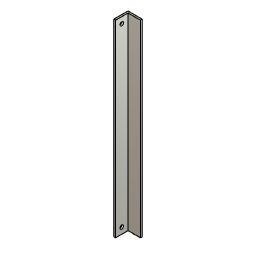
Middle Platform Assembly v15 (Autodesk Fusion 360 archive; units mm, degrees)
design "Angle 336.4 mm 2nd 3rd FR"
Autodesk Fusion 360 part; units mm, degrees
note: some values were not read from the file. Chosen so that the rebuilt part matches the saved one: which bodies a step acts on; a direction. Set by a fixed rule: which sketch regions a step uses.
sketch "Sketch1" plane through (0, 0, 0) normal (0, 1, 0) x (1, 0, 0)
  line L0 (0, -25.4) -> (0, 0)
  line L1 (0, 0) -> (25.4, 0)
  line L2 (12.7, -12.7) -> (11.05, -11.05) construction
  line L3 (3.175, -25.4) -> (3.175, -3.175)
  line L4 (3.175, -3.175) -> (25.4, -3.175)
  line L5 (25.4, -3.175) -> (25.4, 0)
  line L6 (0, -25.4) -> (3.175, -25.4)
  dimension "d1" = 25.4
  dimension "d2" = 25.4
  dimension "d13" = 3.175
  constraint coincident L0.end L2
  constraint coincident L0.end L1.start
  constraint perpendicular L1 L5
  constraint vertical L0
  constraint horizontal L1
  measures "d1" distance of L0.end L1.end
  measures "d2" distance of L0.start L0.end
extrude "Extrude1" add sketch "Sketch1" along normal blind 168.2
hole "Hole3" at (3.175, 157.087, 14.2875) direction (-1, 0, 0) diameter 6.5 end through all
mirror "Mirror1" about plane through (0, 0, 0) normal (0, 1, 0) of bodies 1 merged
equation "d5 = ( 336.4 / 2 ) * 1 mm"
equation "d27 = ( 22.225 / 2 ) * 1 mm"
equation "d19 = 25.4 mm - 11.113 mm"

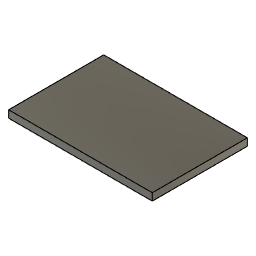
design "Razer 15 inch"
Autodesk Fusion 360 part; units mm, degrees
sketch "Sketch1" plane through (0, 0, 0) normal (0, 0, 1) x (1, 0, 0)
  line L0 (177.5, -117.5) -> (-177.5, -117.5)
  line L1 (-177.5, -117.5) -> (-177.5, 117.5)
  line L2 (-177.5, 117.5) -> (177.5, 117.5)
  line L3 (177.5, 117.5) -> (177.5, -117.5)
  line L4 (177.5, -117.5) -> (-177.5, 117.5) construction
  line L5 (-177.5, -117.5) -> (177.5, 117.5) construction
  dimension "d1" = 355
  dimension "d2" = 235
  constraint horizontal L0
  constraint perpendicular L0 L1
  constraint parallel L0 L2
  constraint parallel L1 L3
  constraint coincident L4 origin
  constraint coincident L5 origin
  measures "d1" distance of L1.end L2.end
  measures "d2" distance of L0.end L1.end
extrude "Extrude1" add sketch "Sketch1" along normal blind 18

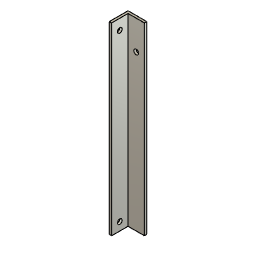
design "Angle 250 mm 1st Standing"
Autodesk Fusion 360 part; units mm, degrees
sketch "Sketch1" plane through (0, 0, 0) normal (0, 1, 0) x (1, 0, 0)
  line L0 (0, -25.4) -> (0, 0)
  line L1 (0, 0) -> (25.4, 0)
  line L2 (12.7, -12.7) -> (11.05, -11.05) construction
  line L3 (3.175, -25.4) -> (3.175, -3.175)
  line L4 (3.175, -3.175) -> (25.4, -3.175)
  line L5 (25.4, -3.175) -> (25.4, 0)
  line L6 (0, -25.4) -> (3.175, -25.4)
  dimension "d1" = 25.4
  dimension "d2" = 25.4
  dimension "d13" = 3.175
  constraint coincident L0.end L2
  constraint coincident L0.end L1.start
  constraint perpendicular L1 L5
  constraint perpendicular L0 L1
  constraint vertical L0
  measures "d1" distance of L0.end L1.end
  measures "d2" distance of L0.start L0.end
extrude "Extrude1" add sketch "Sketch1" along normal blind 250
sketch "Sketch2" plane through (3.175, 0, 0) normal (1, 0, 0) x (0, 0, -1)
  line L0 (-25.4, 0) -> (-3.175, 0)
  line L1 (-3.175, 0) -> (-3.175, 250)
  line L2 (-3.175, 250) -> (-25.4, 250)
  line L3 (-25.4, 250) -> (-25.4, 0)
  circle A0 centre (-14.2875, 235.712) radius 2.76
  circle A1 centre (-14.2875, 11.1125) radius 2.5546
  line L4 (-14.2875, 250) -> (-14.2875, 0) construction
  dimension "d14" = 14.288
  dimension "d15" = 11.1125
  constraint vertical A0.centre A1.centre
  constraint midpoint L2 L4.start
  constraint midpoint L0 L4.end
  constraint coincident A1.centre L4
  measures "d14" distance of L2 A0.centre
  measures "d15" distance of L0 A1.centre
hole "Hole1" at (3.175, 11.1125, 14.2875) at (3.175, 235.712, 14.2875) direction (-1, 0, 0) diameter 6.5 end through all
hole "Hole2" at (14.287, 210.312, 3.175) direction (0, 0, -1) diameter 6.5 end through all
equation "d15 = ( 22.225 / 2 ) * 1 mm"

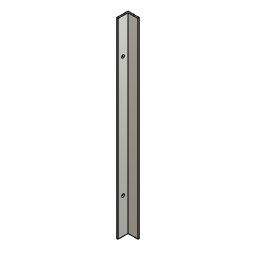
design "Angle 430 mm 2nd Side"
Autodesk Fusion 360 part; units mm, degrees
sketch "Sketch1" plane through (0, 0, 0) normal (0, 1, 0) x (1, 0, 0)
  line L0 (0, -25.4) -> (0, 0)
  line L1 (0, 0) -> (25.4, 0)
  line L2 (12.7, -12.7) -> (11.05, -11.05) construction
  line L3 (3.175, -25.4) -> (3.175, -3.175)
  line L4 (3.175, -3.175) -> (25.4, -3.175)
  line L5 (25.4, -3.175) -> (25.4, 0)
  line L6 (0, -25.4) -> (3.175, -25.4)
  dimension "d1" = 25.4
  dimension "d2" = 25.4
  dimension "d13" = 3.175
  constraint coincident L0.end L2
  constraint coincident L0.end L1.start
  constraint perpendicular L1 L5
  constraint vertical L0
  constraint horizontal L1
  measures "d1" distance of L0.end L1.end
  measures "d2" distance of L0.start L0.end
extrude "Extrude1" add sketch "Sketch1" along normal blind 215
hole "Hole3" at (3.175, 135.512, 14.2875) direction (-1, 0, 0) diameter 6.5 end through all
mirror "Mirror1" about plane through (0, 0, 0) normal (0, 1, 0) of bodies 1 merged
equation "d5 = ( 430 / 2 ) * 1 mm"
equation "d27 = ( 22.225 / 2 ) * 1 mm"
equation "d19 = 25.4 mm - 11.113 mm"

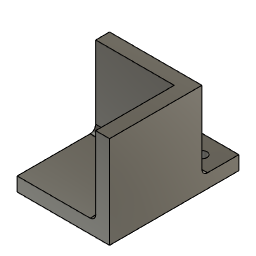
design "Laptop Mount RL/FR"
Autodesk Fusion 360 part; units mm, degrees
sketch "Sketch1" plane through (0, 0, 0) normal (0, 0, 1) x (1, 0, 0)
  line L0 (0, 0) -> (50, 0)
  line L1 (50, 0) -> (50, 50)
  line L2 (0, 7.5) -> (42.5, 7.5)
  line L3 (42.5, 7.5) -> (42.5, 50)
  line L4 (0, 7.5) -> (0, 0)
  line L5 (42.5, 50) -> (50, 50)
  dimension "d1" = -7.5
  dimension "d2" = 50
  dimension "d3" = 50
  constraint coincident L0.start L4.end
  constraint horizontal L0
  constraint perpendicular L0 L1
  constraint perpendicular L2 L4
  constraint perpendicular L1 L5
  measures "d2" distance of L0.start L0.end
  measures "d3" distance of L0.end L1.end
extrude "Extrude1" add sketch "Sketch1" along normal blind 50 makes body 1
sketch "Sketch4" plane through (0, 0, 0) normal (0, 0, 1) x (1, 0, 0)
  line L0 (0, -20) -> (50, -20)
  line L1 (50, -20) -> (50, 50)
  line L2 (50, 50) -> (0, 50)
  line L3 (0, 50) -> (0, -20)
  point P0 (50, 50)
  dimension "d43" = 70
  dimension "d44" = 50
  constraint horizontal L0
  constraint vertical L1
  constraint horizontal L2
  constraint vertical L3
  constraint coincident P0 L1.end
  measures "d43" distance of L0.start L2.end
  measures "d44" distance of P0 L2.end
extrude "Extrude4" add sketch "Sketch4" along normal blind 7.5 bodies 1
sketch "Sketch7" plane through (0, 0, 7.5) normal (0, 0, 1) x (-1, 0, 0)
  line L0 (-50, 20) -> (-50, 0)
  line L1 (0, 0) -> (0, 20)
  line L2 (-50, 0) -> (0, 0)
  line L3 (0, 20) -> (-50, 20)
  point P0 (-10, 10)
  point P1 (-40, 10)
  dimension "d30" = 10
  dimension "d31" = 30
  measures "d30" distance of L1 P0
  measures "d31" distance of P0 P1
hole "Hole1" at (10, -10, 7.5) at (40, -10, 7.5) direction (0, 0, -1) diameter 5.5 depth 10 tip angle 118 bodies 1
ref_plane "WorkPlane1" through (46.25, 50, 25) normal (0, 1, 0) x (-1, 0, 0)
mirror "Mirror1" about plane through (46.25, 50, 25) normal (0, 1, 0) of bodies 1 merged
split "Split1" by plane through (46.25, 50, 25) normal (0, 1, 0) bodies 1 makes body 2 at (29.6023, 69.1741, 0)
fillet "Fillet2" radius 3 3 edges at (25, 100, 7.5) (21.25, 92.5, 7.5) (42.5, 71.25, 7.5) on bodies 2
hidden bodies 1

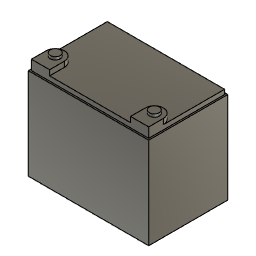
design "Battery"
Autodesk Fusion 360 part; units mm, degrees
sketch "Sketch1" plane through (0, 0, 0) normal (0, 0, 1) x (1, 0, 0)
  line L0 (96, -63) -> (-96, -63)
  line L1 (-96, -63) -> (-96, 63)
  line L2 (-96, 63) -> (96, 63)
  line L3 (96, 63) -> (96, -63)
  line L4 (96, -63) -> (-96, 63) construction
  line L5 (-96, -63) -> (96, 63) construction
  dimension "d1" = 192
  dimension "d2" = 126
  constraint horizontal L0
  constraint perpendicular L0 L1
  constraint parallel L0 L2
  constraint parallel L1 L3
  constraint coincident L4 origin
  constraint coincident L5 origin
  measures "d1" distance of L1.end L2.end
  measures "d2" distance of L0.end L1.end
extrude "Extrude1" add sketch "Sketch1" along normal blind 145.75
sketch "Sketch4" plane through (0, 0, 145.75) normal (0, 0, 1) x (-1, 0, 0)
  line L0 (-96, -63) -> (96, -63)
  line L1 (96, -63) -> (96, 63)
  line L2 (96, 63) -> (-96, 63)
  line L3 (-96, 63) -> (-96, -63)
  line L4 (96, -63) -> (-96, -63)
  line L5 (-96, -63) -> (-96, 63)
  line L6 (-96, 63) -> (96, 63)
  line L7 (96, 63) -> (96, -63)
  line L8 (-93.5, 60.5) -> (93.5, 60.5)
  line L9 (93.5, 60.5) -> (93.5, -60.5)
  line L10 (93.5, -60.5) -> (-93.5, -60.5)
  line L11 (-93.5, -60.5) -> (-93.5, 60.5)
  dimension "d12" = 2.5
  constraint horizontal L4
  constraint vertical L5
  constraint horizontal L6
  constraint vertical L7
  constraint coincident L2.end L3.start
  constraint coincident L0.end L1.start
extrude "Extrude4" add sketch "Sketch4" along normal blind 7.25 contours L8 L9 L10 L11
sketch "Sketch5" plane through (0, 0, 153) normal (0, 0, 1) x (-1, 0, 0)
  line L0 (-93.5, -60.5) -> (93.5, -60.5)
  line L1 (93.5, -60.5) -> (93.5, 60.5)
  line L2 (93.5, 60.5) -> (-93.5, 60.5)
  line L3 (-93.5, 60.5) -> (-93.5, -60.5)
  line L4 (93.5, 60.5) -> (64.5, 60.5)
  line L5 (64.5, 60.5) -> (64.5, 37)
  line L6 (93.5, 37) -> (93.5, 60.5)
  line L7 (-93.5, 60.5) -> (-64.5, 60.5)
  line L8 (-64.5, 60.5) -> (-64.5, 37)
  line L9 (-93.5, 37) -> (-93.5, 60.5)
  arc A0 (64.5, 37) -> (93.5, 37) centre (79, 37) ccw
  arc A1 (-93.5, 37) -> (-64.5, 37) centre (-79, 37) ccw
  dimension "d15" = 14.5
  dimension "d16" = 23.5
  constraint horizontal L4
  constraint vertical L5
  constraint vertical L6
  constraint coincident L1.end L2.start
  constraint horizontal L7
  constraint vertical L8
  constraint vertical L9
  constraint coincident L2.end L3.start
  constraint tangent L6 A0
  constraint tangent L5 A0
  constraint tangent L8 A1
  constraint tangent L9 A1
  constraint equal A0 A1
  constraint equal L5 L8
  measures "d15" radius of A0
  measures "d16" distance of L4.end L5.end
extrude "Extrude5" add sketch "Sketch5" along normal blind 8.5 contours L2 L3 L7 L8 L9 A1 | L1 L2 L4 L5 L6 A0
sketch "Sketch6" plane through (0, 0, 161.5) normal (0, 0, 1) x (-1, 0, 0)
  arc A0 (64.5, 37) -> (93.5, 37) centre (79, 37) ccw
  line L0 (93.5, 37) -> (93.5, 60.5)
  line L1 (93.5, 60.5) -> (64.5, 60.5)
  line L2 (64.5, 60.5) -> (64.5, 37)
  circle A1 centre (79, 37) radius 8
  circle A2 centre (-79, 37) radius 8
  arc A3 (-93.5, 37) -> (-64.5, 37) centre (-79, 37) ccw
  dimension "d19" = 16
  constraint concentric A0 A1
  constraint concentric A2 A3
  constraint equal A1 A2
  measures "d19" diameter of A1
extrude "Extrude6" add sketch "Sketch6" along normal blind 4.6 contours A1 | A2
equation "d3 = 153 mm - 7.25 mm"
equation "d16 = 38 mm - 14.5 mm"

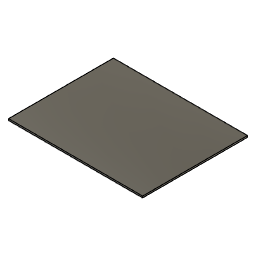
design "2nd Plate M"
Autodesk Fusion 360 part; units mm, degrees
sketch "Sketch1" plane through (0, 0, 0) normal (0, 0, 1) x (1, 0, 0)
  line L0 (-250, 225) -> (180, 225)
  line L1 (180, 225) -> (180, -111.4)
  line L2 (180, -111.4) -> (-250, -111.4)
  line L3 (-250, -111.4) -> (-250, 225)
  dimension "d1" = 336.4
  dimension "d2" = 430
  constraint horizontal L0
  constraint vertical L1
  constraint horizontal L2
  constraint vertical L3
  measures "d1" distance of L0.start L2.end
  measures "d2" distance of L0.start L0.end
extrude "Extrude1" add sketch "Sketch1" along normal blind 5

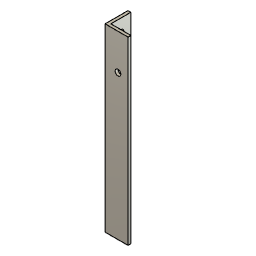
design "Angle 200 mm 2nd Standing Reverse"
Autodesk Fusion 360 part; units mm, degrees
sketch "Sketch1" plane through (0, 0, 0) normal (0, 1, 0) x (1, 0, 0)
  line L0 (0, -25.4) -> (0, 0)
  line L1 (0, 0) -> (25.4, 0)
  line L2 (12.7, -12.7) -> (11.05, -11.05) construction
  line L3 (3.175, -25.4) -> (3.175, -3.175)
  line L4 (3.175, -3.175) -> (25.4, -3.175)
  line L5 (25.4, -3.175) -> (25.4, 0)
  line L6 (0, -25.4) -> (3.175, -25.4)
  dimension "d1" = 25.4
  dimension "d2" = 25.4
  dimension "d13" = 3.175
  constraint coincident L0.end L2
  constraint coincident L0.end L1.start
  constraint perpendicular L1 L5
  constraint vertical L0
  constraint horizontal L1
  measures "d1" distance of L0.end L1.end
  measures "d2" distance of L0.start L0.end
extrude "Extrude1" add sketch "Sketch1" along normal blind 200 makes body 1
hole "Hole3" at (3.175, 11.113, 14.287) direction (-1, 0, 0) diameter 6.5 end through all bodies 1
hole "Hole4" at (3.175, 185.772, 14.287) direction (-1, 0, 0) diameter 6.5 depth 30 tip angle 118 bodies 1
hole "Hole5" at (14.287, 160.312, 3.175) direction (0, 0, -1) diameter 6.5 depth 30 tip angle 118 bodies 1
mirror "Mirror2" about plane through (0, 0, 0) normal (0, 0, -1) of bodies 1 makes body 2
delete_body "RemoveBody1" bodies 1

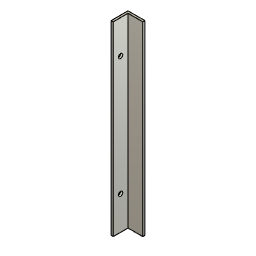
design "Angle 280 mm Battery Holder"
Autodesk Fusion 360 part; units mm, degrees
sketch "Sketch1" plane through (0, 0, 0) normal (0, 1, 0) x (1, 0, 0)
  line L0 (0, -25.4) -> (0, 0)
  line L1 (0, 0) -> (25.4, 0)
  line L2 (12.7, -12.7) -> (11.05, -11.05) construction
  line L3 (3.175, -25.4) -> (3.175, -3.175)
  line L4 (3.175, -3.175) -> (25.4, -3.175)
  line L5 (25.4, -3.175) -> (25.4, 0)
  line L6 (0, -25.4) -> (3.175, -25.4)
  dimension "d1" = 25.4
  dimension "d2" = 25.4
  dimension "d13" = 3.175
  constraint coincident L0.end L2
  constraint coincident L0.end L1.start
  constraint perpendicular L1 L5
  constraint vertical L0
  constraint horizontal L1
  measures "d1" distance of L0.end L1.end
  measures "d2" distance of L0.start L0.end
extrude "Extrude1" add sketch "Sketch1" along normal blind 139.6
hole "Hole3" at (3.175, 89.6, 14.2875) direction (-1, 0, 0) diameter 6.5 end through all
mirror "Mirror1" about plane through (0, 0, 0) normal (0, 1, 0) of bodies 1 merged
equation "d5 = ( 279.2 / 2 ) * 1 mm"
equation "d27 = ( 22.225 / 2 ) * 1 mm"
equation "d19 = 25.4 mm - 11.113 mm"

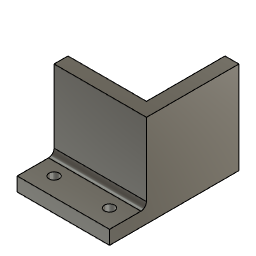
design "Laptop Mount FL/RR"
Autodesk Fusion 360 part; units mm, degrees
sketch "Sketch1" plane through (0, 0, 0) normal (0, 0, 1) x (1, 0, 0)
  line L0 (0, 0) -> (50, 0)
  line L1 (50, 0) -> (50, 50)
  line L2 (0, 7.5) -> (42.5, 7.5)
  line L3 (42.5, 7.5) -> (42.5, 50)
  line L4 (0, 7.5) -> (0, 0)
  line L5 (42.5, 50) -> (50, 50)
  dimension "d1" = -7.5
  dimension "d2" = 50
  dimension "d3" = 50
  constraint coincident L0.start L4.end
  constraint horizontal L0
  constraint perpendicular L0 L1
  constraint perpendicular L2 L4
  constraint perpendicular L1 L5
  measures "d2" distance of L0.start L0.end
  measures "d3" distance of L0.end L1.end
extrude "Extrude1" add sketch "Sketch1" along normal blind 50
sketch "Sketch4" plane through (0, 0, 0) normal (0, 0, 1) x (1, 0, 0)
  line L0 (50, -20) -> (0, -20)
  line L1 (0, -20) -> (0, 50)
  line L2 (0, 50) -> (50, 50)
  line L3 (50, 50) -> (50, -20)
  point P0 (50, 50)
  dimension "d43" = 70
  dimension "d44" = 50
  constraint horizontal L0
  constraint vertical L1
  constraint horizontal L2
  constraint vertical L3
  constraint coincident P0 L2.end
  measures "d43" distance of L0.end L1.end
  measures "d44" distance of L1.end P0
extrude "Extrude4" add sketch "Sketch4" along normal blind 7.5
sketch "Sketch7" plane through (0, 0, 7.5) normal (0, 0, 1) x (-1, 0, 0)
  line L0 (0, 0) -> (0, 20)
  line L1 (-50, 0) -> (0, 0)
  line L2 (0, 20) -> (-50, 20)
  line L3 (-50, 20) -> (-50, 0)
  point P0 (-10, 10)
  point P1 (-40, 10)
  dimension "d35" = 30
  measures "d35" distance of P0 P1
hole "Hole1" at (10, -10, 7.5) at (40, -10, 7.5) direction (0, 0, -1) diameter 5.5 depth 10 tip angle 118
fillet "Fillet1" radius 3 1 edges at (25, 0, 7.5)
fillet "Fillet1" radius 3 2 edges at (21.25, 7.5, 7.5) (42.5, 28.75, 7.5)

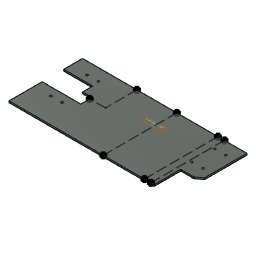
design "Metal Board"
Autodesk Fusion 360 part; units mm, degrees
sketch "Sketch1" plane through (0, 0, 0) normal (0, 0, 1) x (1, 0, 0)
  line L0 (0, 0) -> (680, 0)
  line L1 (680, 0) -> (680, -304)
  line L2 (680, -304) -> (0, -304)
  line L3 (0, -304) -> (0, 0)
  dimension "d1" = 680
  dimension "d2" = 304
  constraint horizontal L0
  constraint vertical L1
  constraint horizontal L2
  constraint vertical L3
  constraint coincident L0.start L3.end
  measures "d1" distance of L0.start L0.end
  measures "d2" distance of L0.start L2.end
extrude "Extrude1" add sketch "Sketch1" along normal blind 6.25
sketch "Sketch2" plane through (0, 0, 6.25) normal (0, 0, 1) x (-1, 0, 0)
  line L0 (0, 304) -> (-680, 304)
  line L1 (-680, 304) -> (-680, 0)
  line L2 (-680, 0) -> (0, 0)
  line L3 (0, 0) -> (0, 304)
  line L4 (-160, 120) -> (-160, 167)
  line L5 (-160, 167) -> (0, 167)
  line L6 (0, 167) -> (0, 78)
  line L7 (-120, 78) -> (-120, 120)
  line L8 (-120, 120) -> (-160, 120)
  line L9 (-120, 78) -> (0, 78)
  line L10 (-680, 304) -> (-600, 304)
  line L11 (-600, 304) -> (-600, 194)
  line L12 (-600, 194) -> (-655, 194)
  line L13 (-680, 175) -> (-680, 304)
  line L14 (-655, 194) -> (-680, 175)
  dimension "d10" = 120
  dimension "d11" = 42
  dimension "d12" = 47
  dimension "d13" = 120
  dimension "d14" = 160
  dimension "d15" = 110
  dimension "d19" = 129
  dimension "d20" = 55
  dimension "d21" = 80
  constraint vertical L4
  constraint horizontal L5
  constraint coincident L3 L6.end
  constraint perpendicular L5 L6
  constraint perpendicular L5 L7
  constraint perpendicular L7 L8
  constraint coincident L4.start L8.end
  constraint perpendicular L6 L9
  constraint horizontal L10
  constraint vertical L11
  constraint horizontal L12
  constraint vertical L13
  constraint coincident L0.end L1.start
  measures "d10" distance of L6.end L7.start
  measures "d11" distance of L7.start L7.end
  measures "d12" distance of L4.start L4.end
  measures "d13" distance of L2 L8
  measures "d14" distance of L4.end L5.end
  measures "d15" distance of L10.end L11.end
  measures "d19" distance of L0.end L13.start
  measures "d20" distance of L11.end L12.end
  measures "d21" distance of L0.end L10.end
extrude "Extrude3" cut sketch "Sketch2" against normal blind 6.25 contours L0 L1 L10 L11 L12 L13 L14 | L3 L4 L5 L6 L7 L8 L9
sketch "Sketch4" plane through (0, 0, 6.25) normal (0, 0, 1) x (-1, 0, 0)
  line L0 (-160, 167) -> (0, 167)
  line L1 (0, 167) -> (0, 304)
  line L2 (0, 304) -> (-600, 304)
  line L3 (-600, 304) -> (-600, 194)
  line L4 (-600, 194) -> (-655, 194)
  line L5 (-655, 194) -> (-680, 175)
  line L6 (-680, 175) -> (-680, 0)
  line L7 (-680, 0) -> (0, 0)
  line L8 (0, 0) -> (0, 78)
  line L9 (0, 78) -> (-120, 78)
  line L10 (-120, 78) -> (-120, 120)
  line L11 (-120, 120) -> (-160, 120)
  line L12 (-160, 120) -> (-160, 167)
  line L13 (-69, 200) -> (-115, 200) construction
  line L14 (-597, 145) -> (-643, 145) construction
  line L15 (-115, 50) -> (-69, 50) construction
  line L16 (-597, 50) -> (-643, 50) construction
  point P0 (-643, 145)
  point P1 (-597, 145)
  point P2 (-115, 200)
  point P3 (-69, 200)
  point P4 (-115, 50)
  point P5 (-69, 50)
  point P6 (-597, 50)
  point P7 (-643, 50)
  dimension "d33" = 46
  dimension "d35" = 150
  dimension "d36" = 50
  dimension "d37" = 95
  dimension "d38" = 115
  dimension "d44" = 83
  constraint horizontal P2 P3
  constraint horizontal P0 P1
  constraint coincident P3 L13.start
  constraint coincident P2 L13.end
  constraint parallel L7 L13
  constraint coincident P1 L14.start
  constraint coincident P0 L14.end
  constraint equal L13 L14
  constraint horizontal P4 P5
  constraint horizontal P5 P6
  constraint horizontal P6 P7
  constraint vertical P1 P6
  constraint coincident P4 L15.start
  constraint coincident P5 L15.end
  constraint coincident P6 L16.start
  constraint coincident P7 L16.end
  constraint equal L14 L16
  constraint equal L13 L15
  constraint vertical P2 P4
  constraint collinear L15 L16
  measures "d33" distance of P6 P7
  measures "d35" distance of P2 P4
  measures "d36" distance of L7 P4
  measures "d37" distance of P1 P6
  measures "d38" distance of L8 P4
  measures "d44" distance of L6 P6
hole "Hole2" at (597, -145, 6.25) at (643, -145, 6.25) at (115, -200, 6.25) at (69, -200, 6.25) at (115, -50, 6.25) at (69, -50, 6.25) at (643, -50, 6.25) at (597, -50, 6.25) direction (0, 0, -1) diameter 8.5 depth 6.25 tip angle 118
sketch "Sketch5" plane through (0, 0, 6.25) normal (0, 0, 1) x (-1, 0, 0)
  circle A0 centre (-643, 50) radius 4.25
  circle A1 centre (-115, 50) radius 4.25
  circle A2 centre (-115, 200) radius 4.25
  circle A3 centre (-597, 145) radius 4.25
  circle A4 centre (-643, 145) radius 4.25
  circle A5 centre (-69, 200) radius 4.25
  circle A6 centre (-69, 50) radius 4.25
  circle A7 centre (-597, 50) radius 4.25
  line L0 (-160, 167) -> (0, 167)
  line L1 (0, 167) -> (0, 304)
  line L2 (0, 304) -> (-600, 304)
  line L3 (-600, 304) -> (-600, 194)
  line L4 (-600, 194) -> (-655, 194)
  line L5 (-655, 194) -> (-680, 175)
  line L6 (-680, 175) -> (-680, 0)
  line L7 (-680, 0) -> (0, 0)
  line L8 (0, 0) -> (0, 78)
  line L9 (0, 78) -> (-120, 78)
  line L10 (-120, 78) -> (-120, 120)
  line L11 (-120, 120) -> (-160, 120)
  line L12 (-160, 120) -> (-160, 167)
  line L13 (-225, 0) -> (-225, 130) construction
  line L14 (-587, 0) -> (-587, 304) construction
  line L15 (-390, 0) -> (-390, 304) construction
  line L16 (-225, 130) -> (-160, 130) construction
  line L17 (-347.9611, 97.8111) -> (-427.9611, 97.8111) construction
  line L18 (-427.9611, 97.8111) -> (-427.9611, 77.8111) construction
  line L19 (-427.9611, 77.8111) -> (-347.9611, 77.8111) construction
  line L20 (-347.9611, 77.8111) -> (-347.9611, 97.8111) construction
  line L21 (-560, 0) -> (-560, 304) construction
  dimension "d39" = 225
  dimension "d41" = 390
  dimension "d42" = 130
  dimension "d43" = 10
  dimension "d46" = 170
  dimension "d47" = 93
  constraint coincident L7 L13.start
  constraint perpendicular L2 L13
  constraint coincident L7 L14.start
  constraint coincident L2 L14.end
  constraint perpendicular L2 L14
  constraint coincident L7 L15.start
  constraint coincident L2 L15.end
  constraint perpendicular L2 L15
  constraint coincident L12 L16.end
  constraint perpendicular L12 L16
  constraint coincident L7 L21.start
  constraint coincident L2 L21.end
  constraint perpendicular L2 L21
  measures "d39" distance of L8 L13
  measures "d41" distance of L1 L15
  measures "d42" distance of L7 L16
  measures "d46" distance of L15 L21
  measures "d47" distance of L6 L14
equation "d19 = 304 mm - 175 mm"

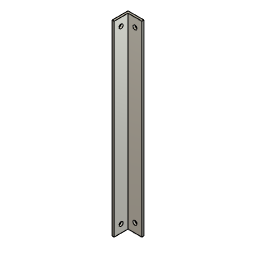
design "Angle 300 mm Base Side"
Autodesk Fusion 360 part; units mm, degrees
sketch "Sketch1" plane through (0, 0, 0) normal (0, 1, 0) x (1, 0, 0)
  line L0 (0, -25.4) -> (0, 0)
  line L1 (0, 0) -> (25.4, 0)
  line L2 (12.7, -12.7) -> (11.05, -11.05) construction
  line L3 (3.175, -25.4) -> (3.175, -3.175)
  line L4 (3.175, -3.175) -> (25.4, -3.175)
  line L5 (25.4, -3.175) -> (25.4, 0)
  line L6 (0, -25.4) -> (3.175, -25.4)
  dimension "d1" = 25.4
  dimension "d2" = 25.4
  dimension "d13" = 3.175
  constraint coincident L0.end L2
  constraint coincident L0.end L1.start
  constraint perpendicular L1 L5
  constraint vertical L0
  constraint horizontal L1
  measures "d1" distance of L0.end L1.end
  measures "d2" distance of L0.start L0.end
extrude "Extrude1" add sketch "Sketch1" along normal blind 300
sketch "Sketch2" plane through (3.175, 0, 0) normal (1, 0, 0) x (0, 0, -1)
  line L0 (-25.4, 0) -> (-3.175, 0)
  line L1 (-3.175, 0) -> (-3.175, 300)
  line L2 (-3.175, 300) -> (-25.4, 300)
  line L3 (-25.4, 300) -> (-25.4, 0)
  circle A0 centre (-14.2875, 287.3) radius 2.76
  circle A1 centre (-14.2875, 12.7) radius 2.5546
  line L4 (-14.2875, 300) -> (-14.2875, 0) construction
  dimension "d14" = 12.7
  dimension "d15" = 12.7
  constraint vertical A0.centre A1.centre
  constraint midpoint L2 L4.start
  constraint midpoint L0 L4.end
  constraint coincident A1.centre L4
  measures "d14" distance of L2 A0.centre
  measures "d15" distance of L0 A1.centre
hole "Hole1" at (3.175, 12.7, 14.2875) at (3.175, 287.3, 14.2875) direction (-1, 0, 0) diameter 6.5 end through all
sketch "Sketch3" plane through (0, 0, 3.175) normal (0, 0, 1) x (1, 0, 0)
  line L0 (3.175, 0) -> (25.4, 0)
  line L1 (25.4, 0) -> (25.4, 300)
  line L2 (25.4, 300) -> (3.175, 300)
  line L3 (3.175, 300) -> (3.175, 0)
  line L4 (14.2875, 0) -> (14.2875, 300) construction
  circle A0 centre (14.2875, 285.713) radius 2.8949
  circle A1 centre (14.2875, 14.287) radius 4.0168
  dimension "d19" = 14.287
  dimension "d20" = 14.287
  constraint midpoint L0 L4.start
  constraint midpoint L2 L4.end
  constraint coincident L4 A0.centre
  constraint coincident L4 A1.centre
  measures "d19" distance of L4.end A0.centre
  measures "d20" distance of L4.start A1.centre
hole "Hole2" at (14.2875, 14.287, 3.175) at (14.2875, 285.713, 3.175) direction (0, 0, -1) diameter 6.5 end through all
equation "d14 = ( 25.4 / 2 ) * 1 mm"
equation "d15 = ( 25.4 / 2 ) * 1 mm"
equation "d19 = 25.4 mm - 11.113 mm"

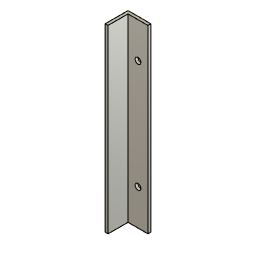
design "Angle 200 mm 2nd Side"
Autodesk Fusion 360 part; units mm, degrees
sketch "Sketch1" plane through (0, 0, 0) normal (0, 1, 0) x (1, 0, 0)
  line L0 (0, -25.4) -> (0, 0)
  line L1 (0, 0) -> (25.4, 0)
  line L2 (12.7, -12.7) -> (11.05, -11.05) construction
  line L3 (3.175, -25.4) -> (3.175, -3.175)
  line L4 (3.175, -3.175) -> (25.4, -3.175)
  line L5 (25.4, -3.175) -> (25.4, 0)
  line L6 (0, -25.4) -> (3.175, -25.4)
  dimension "d1" = 25.4
  dimension "d2" = 25.4
  dimension "d13" = 3.175
  constraint coincident L0.end L2
  constraint coincident L0.end L1.start
  constraint perpendicular L1 L5
  constraint perpendicular L0 L1
  constraint vertical L0
  measures "d1" distance of L0.end L1.end
  measures "d2" distance of L0.start L0.end
extrude "Extrude1" add sketch "Sketch1" along normal blind 100.4
hole "Hole3" at (14.2875, 60.7125, 3.175) direction (0, 0, -1) diameter 6.5 depth 30 tip angle 118
mirror "Mirror2" about plane through (0, 0, 0) normal (0, -1, 0) of bodies 1 merged
equation "d29 = ( 22.225 / 2 ) * 1 mm"
equation "d30 = ( 22.225 / 2 ) * 1 mm + 25.4 mm + 3.175 mm"

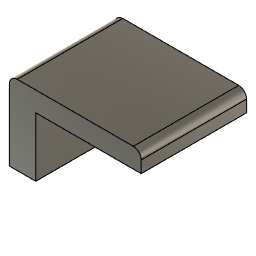
design "Laptop Hold Vertical"
Autodesk Fusion 360 part; units mm, degrees
sketch "Sketch1" plane through (0, 0, 0) normal (0, 1, 0) x (1, 0, 0)
  line L0 (0, 0) -> (0, -30)
  line L1 (0, -30) -> (50, -30)
  line L2 (50, -30) -> (50, -22.5)
  line L3 (50, -22.5) -> (10, -22.5)
  line L4 (10, -22.5) -> (10, 0)
  line L5 (10, 0) -> (0, 0)
  dimension "d1" = 10
  dimension "d2" = 30
  dimension "d3" = 50
  dimension "d9" = 7.5
  constraint coincident L0.start L5.end
  constraint vertical L0
  constraint perpendicular L0 L1
  constraint perpendicular L1 L2
  constraint perpendicular L2 L3
  constraint perpendicular L3 L4
  constraint perpendicular L0 L5
  measures "d1" distance of L4.end L0.start
  measures "d2" distance of L0.start L0.end
  measures "d3" distance of L0.end L1.end
  measures "d9" distance of L1.end L2.end
extrude "Extrude1" add sketch "Sketch1" along normal blind 40
sketch "Sketch2" plane through (10, 0, 0) normal (1, 0, 0) x (0, 1, 0)
  line L0 (0, 22.5) -> (0, 0)
  line L1 (0, 0) -> (40, 0)
  line L2 (40, 0) -> (40, 22.5)
  line L3 (40, 22.5) -> (0, 22.5)
  line L4 (23.25, 15) -> (23.25, 7.5)
  line L5 (16.75, 7.5) -> (16.75, 15)
  arc A0 (23.25, 15) -> (16.75, 15) centre (20, 15) ccw
  arc A1 (16.75, 7.5) -> (23.25, 7.5) centre (20, 7.5) ccw
  line L6 (0, 0) -> (40, 22.5) construction
  line L7 (20, 15) -> (20, 7.5) construction
  dimension "d6" = 6.5
  dimension "d7" = 7.5
  constraint vertical L4
  constraint vertical L5
  constraint tangent L5 A0
  constraint tangent L5 A1
  constraint tangent L4 A1
  constraint tangent L4 A0
  constraint coincident L0.end L1.start
  constraint coincident L2.end L3.start
  constraint coincident A0.centre L7.start
  constraint coincident A1.centre L7.end
  constraint midpoint L6 L7
  measures "d6" distance of L4 L5
  measures "d7" distance of L4.start L4.end
extrude "Extrude2" cut sketch "Sketch2" against normal through all contours L4 L5 A0 A1
fillet "Fillet1" radius 3 2 edges at (0, 20, 30) (50, 20, 30)

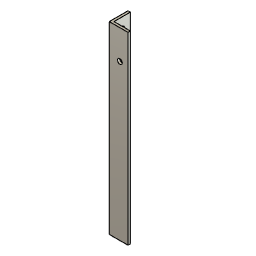
design "Angle 250 mm 1st Standing Reverse"
Autodesk Fusion 360 part; units mm, degrees
sketch "Sketch1" plane through (0, 0, 0) normal (0, 1, 0) x (1, 0, 0)
  line L0 (0, -25.4) -> (0, 0)
  line L1 (0, 0) -> (25.4, 0)
  line L2 (12.7, -12.7) -> (11.05, -11.05) construction
  line L3 (3.175, -25.4) -> (3.175, -3.175)
  line L4 (3.175, -3.175) -> (25.4, -3.175)
  line L5 (25.4, -3.175) -> (25.4, 0)
  line L6 (0, -25.4) -> (3.175, -25.4)
  dimension "d1" = 25.4
  dimension "d2" = 25.4
  dimension "d13" = 3.175
  constraint coincident L0.end L2
  constraint coincident L0.end L1.start
  constraint perpendicular L1 L5
  constraint perpendicular L0 L1
  constraint vertical L0
  measures "d1" distance of L0.end L1.end
  measures "d2" distance of L0.start L0.end
extrude "Extrude1" add sketch "Sketch1" along normal blind 250 makes body 1
sketch "Sketch2" plane through (3.175, 0, 0) normal (1, 0, 0) x (0, 0, -1)
  line L0 (-25.4, 0) -> (-3.175, 0)
  line L1 (-3.175, 0) -> (-3.175, 250)
  line L2 (-3.175, 250) -> (-25.4, 250)
  line L3 (-25.4, 250) -> (-25.4, 0)
  circle A0 centre (-14.2875, 235.712) radius 2.76
  circle A1 centre (-14.2875, 11.1125) radius 2.5546
  line L4 (-14.2875, 250) -> (-14.2875, 0) construction
  dimension "d14" = 14.288
  dimension "d15" = 11.1125
  constraint vertical A0.centre A1.centre
  constraint midpoint L2 L4.start
  constraint midpoint L0 L4.end
  constraint coincident A1.centre L4
  measures "d14" distance of L2 A0.centre
  measures "d15" distance of L0 A1.centre
hole "Hole1" at (3.175, 11.1125, 14.2875) at (3.175, 235.712, 14.2875) direction (-1, 0, 0) diameter 6.5 end through all bodies 1
mirror "Mirror1" about plane through (0, 0, 0) normal (0, 0, 1) of bodies 1 merged
split "Split1" by plane through (0, 0, 0) normal (0, 0, 1) bodies 1 makes body 2 at (0, 161.2807, 3.8764)
delete_body "RemoveBody1" bodies 2
hole "Hole2" at (14.287, 210.312, -3.175) direction (0, 0, 1) diameter 6.5 depth 3.175 tip angle 118 bodies 1
equation "d15 = ( 22.225 / 2 ) * 1 mm"

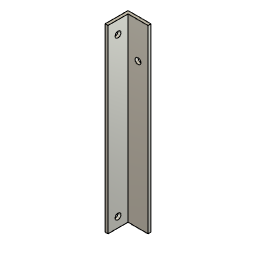
design "Angle 200 mm 2nd Standing"
Autodesk Fusion 360 part; units mm, degrees
sketch "Sketch1" plane through (0, 0, 0) normal (0, 1, 0) x (1, 0, 0)
  line L0 (0, -25.4) -> (0, 0)
  line L1 (0, 0) -> (25.4, 0)
  line L2 (12.7, -12.7) -> (11.05, -11.05) construction
  line L3 (3.175, -25.4) -> (3.175, -3.175)
  line L4 (3.175, -3.175) -> (25.4, -3.175)
  line L5 (25.4, -3.175) -> (25.4, 0)
  line L6 (0, -25.4) -> (3.175, -25.4)
  dimension "d1" = 25.4
  dimension "d2" = 25.4
  dimension "d13" = 3.175
  constraint coincident L0.end L2
  constraint coincident L0.end L1.start
  constraint perpendicular L1 L5
  constraint vertical L0
  constraint horizontal L1
  measures "d1" distance of L0.end L1.end
  measures "d2" distance of L0.start L0.end
extrude "Extrude1" add sketch "Sketch1" along normal blind 200
hole "Hole3" at (3.175, 11.113, 14.287) direction (-1, 0, 0) diameter 6.5 end through all
hole "Hole4" at (3.175, 185.772, 14.287) direction (-1, 0, 0) diameter 6.5 depth 30 tip angle 118
hole "Hole5" at (14.287, 160.312, 3.175) direction (0, 0, -1) diameter 6.5 depth 30 tip angle 118

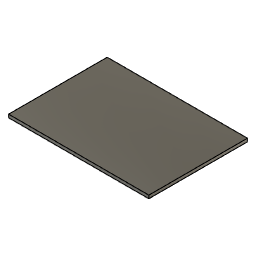
design "3rd Plate M"
Autodesk Fusion 360 part; units mm, degrees
sketch "Sketch1" plane through (0, 0, 0) normal (0, 0, 1) x (1, 0, 0)
  line L0 (142.8, -100.4) -> (-142.8, -100.4)
  line L1 (-142.8, -100.4) -> (-142.8, 100.4)
  line L2 (-142.8, 100.4) -> (142.8, 100.4)
  line L3 (142.8, 100.4) -> (142.8, -100.4)
  line L4 (142.8, -100.4) -> (-142.8, 100.4) construction
  line L5 (-142.8, -100.4) -> (142.8, 100.4) construction
  dimension "d1" = 200.8
  dimension "d2" = 285.6
  constraint horizontal L0
  constraint perpendicular L0 L1
  constraint parallel L0 L2
  constraint parallel L1 L3
  constraint coincident L4 origin
  constraint coincident L5 origin
  measures "d1" distance of L0.end L1.end
  measures "d2" distance of L1.end L2.end
extrude "Extrude1" add sketch "Sketch1" along normal blind 6.35
